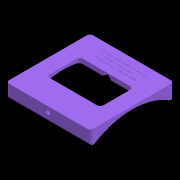
# Autodesk Inventor part: controls_flat
Saved by Autodesk Inventor 2020.2 (Build 242310000, 310)
## iProperties
Created: 2020-04-29
Part Number: controls_flat
Material: PC/ABS Plastic
Document SubType Name: Modeling
Designer: agmlego
Mass: 56.1981 g
Surface Area: 381.586 cm^2
Volume: 157.298 cm^3
Density: 0.357273 g/cm^3
Appearance: Violet
Author: agmlego
Autodesk Inventor part; units mm, degrees
(part 1 of 3)
ref_plane "YZ Plane" through (0, 0, 0) normal (1, 0, 0) x (0, 1, 0)
ref_plane "XZ Plane" through (0, 0, 0) normal (0, 1, 0) x (-1, 0, 0)
ref_plane "XY Plane" through (0, 0, 0) normal (0, 0, 1) x (1, 0, 0)
sketch "Sketch1" plane through (0, 0, 0) normal (1, 0, 0) x (0, 1, 0)
  arc A0 (87.9555, -65.2863) -> (87.9555, 65.2863) centre (0, 0) ccw
  line L0 (113.8555, 20.8363) -> (107.5375, 20.8363) construction
  line L1 (107.5375, 20.8363) -> (107.5375, -20.8363) construction
  line L2 (107.5375, -20.8363) -> (113.8555, -20.8363) construction
  line L3 (113.8555, -20.8363) -> (113.8555, 20.8363) construction
  line L4 (113.8555, 65.2863) -> (87.9555, 65.2863)
  line L5 (87.9555, -65.2863) -> (113.8555, -65.2863)
  line L6 (113.8555, -65.2863) -> (113.8555, 65.2863)
  point P0 (113.8555, 0)
  dimension "d0" = 219.075
  dimension "d1" = 113.8555
  dimension "d2" = 107.5375
  dimension "d3" = 44.45
  constraints: 14 end point, 4 parallel, 4 point on circle, 2 horizontal, 2 midpoint, 1 centre point, 1 coincident, 1 perpendicular
  measures "d0" diameter of A0
  measures "d1" distance from line of L3 A0.centre
  measures "d2" distance from line of A0.centre L1
  measures "d3" distance between parallel lines of L4 L0
extrude "Extrusion1" add sketch "Sketch1" along normal blind 130.8
sketch "Sketch2" plane through (0, 113.8555, 65.2863) normal (0, 1, 0) x (1, 0, 0)
  line L0 (25.4, 44.4498) -> (105.4, 44.4498) construction
  line L1 (105.4, 44.4498) -> (105.4, 86.1228) construction
  line L2 (105.4, 86.1228) -> (25.4, 86.1228) construction
  line L3 (25.4, 86.1228) -> (25.4, 44.4498) construction
  line L4 (0, 130.5725) -> (0, 0) construction
  circle A0 centre (28.575, 44.4498) radius 3.175 construction
  circle A1 centre (28.575, 44.4498) radius 4.953 construction
  line L5 (23.622, 39.4968) -> (107.178, 39.4968)
  line L6 (107.178, 39.4968) -> (107.178, 91.0758)
  line L7 (107.178, 91.0758) -> (23.622, 91.0758)
  line L8 (23.622, 91.0758) -> (23.622, 39.4968)
  point P0 (0, 65.2863)
  point P1 (25.4, 65.2863)
  point P2 (0, 65.2863)
  point P3 (23.622, 65.2863)
  point P4 (65.4, 91.0758)
  point P5 (65.4, 86.1228)
  dimension "d6" = 80
  dimension "d7" = 25.4
  dimension "d8" = 41.673
  dimension "d9" = 6.35
  dimension "d10" = 9.906
  constraints: 16 end point, 5 midpoint, 4 parallel, 3 tangent, 2 centre point, 2 horizontal, 2 horizontal alignment, 2 perpendicular, 1 coincident, 1 point on line, 1 vertical alignment
  measures "d6" distance of L1.end L2.end
  measures "d7" distance between parallel lines of L4 L3
  measures "d8" distance of L0.end L1.end
  measures "d9" diameter of A0
  measures "d10" diameter of A1
extrude "Extrusion2" cut sketch "Sketch2" against normal through all
fillet "Fillet1" radius 4.953 10 edges at (23.622, 110.1569, -25.7895) (23.622, 110.1569, 25.7895) (107.178, 110.1569, 25.7895) (107.178, 110.1569, -25.7895) (65.4, 87.9555, 65.2863) (65.4, 87.9555, -65.2863) (0, 100.9055, 65.2863) (0, 100.9055, -65.2863) (130.8, 100.9055, -65.2863) (130.8, 100.9055, 65.2863)
sketch "Sketch3" plane through (0, 113.8555, 65.2863) normal (0, 1, 0) x (1, 0, 0)
  line L0 (16.3484, 118.3923) -> (114.0865, 118.3923) construction
  line L1 (114.0865, 118.3923) -> (114.0865, 82.237) construction
  line L2 (114.0865, 82.237) -> (16.3484, 82.237) construction
  line L3 (16.3484, 82.237) -> (16.3484, 118.3923) construction
  spline S0 degree 2 poles (32.4092, 115.5523) (32.2458, 115.4201) (31.849, 115.3086) (31.6104, 115.3086) knots 0 0 0 1 2 2 2
  spline S1 degree 2 poles (31.6104, 115.3086) (31.3225, 115.3086) (30.8609, 115.5601) (30.5393, 115.9881) (30.3707, 116.5638) (30.3707, 116.888) knots 0 0 0 1 2 3 4 4 4
  spline S2 degree 2 poles (30.3707, 116.888) (30.3707, 117.1915) (30.5237, 117.7361) (30.8401, 118.1459) (31.3251, 118.3871) (31.6571, 118.3871) knots 0 0 0 1 2 3 4 4 4
  spline S3 degree 2 poles (31.6571, 118.3871) (31.8879, 118.3871) (32.3003, 118.2393) (32.4455, 118.1018) knots 0 0 0 1 2 2 2
  line L4 (32.4455, 118.1018) -> (32.264, 117.8865)
  spline S4 degree 2 poles (32.264, 117.8865) (32.168, 117.9514) (31.8775, 118.0473) (31.6908, 118.0473) knots 0 0 0 1 2 2 2
  spline S5 degree 2 poles (31.6908, 118.0473) (31.4444, 118.0473) (31.1047, 117.8632) (30.8868, 117.5468) (30.7883, 117.1292) (30.7883, 116.8932) knots 0 0 0 1 2 3 4 4 4
  spline S6 degree 2 poles (30.7883, 116.8932) (30.7883, 116.7557) (30.8323, 116.4653) (30.9231, 116.1878) (31.0658, 115.944) (31.2603, 115.7598) (31.5093, 115.6509) (31.6623, 115.6509) knots 0 0 0 1 2 3 4 5 6 6 6
  spline S7 degree 2 poles (31.6623, 115.6509) (31.7531, 115.6509) (31.9035, 115.6665) (32.0409, 115.7028) (32.1784, 115.7624) (32.2562, 115.8065) knots 0 0 0 1 2 3 4 4 4
  line L5 (32.2562, 115.8065) -> (32.4092, 115.5523)
  spline S8 degree 2 poles (34.2065, 115.3086) (33.8901, 115.3086) (33.387, 115.542) (33.0369, 115.9518) (32.8501, 116.5171) (32.8501, 116.8491) knots 0 0 0 1 2 3 4 4 4
  spline S9 degree 2 poles (32.8501, 116.8491) (32.8501, 117.1785) (33.0317, 117.7439) (33.3766, 118.1537) (33.8823, 118.3871) (34.2065, 118.3871) knots 0 0 0 1 2 3 4 4 4
  spline S10 degree 2 poles (34.2065, 118.3871) (34.5204, 118.3871) (35.0261, 118.1537) (35.3762, 117.7439) (35.563, 117.1785) (35.563, 116.8491) knots 0 0 0 1 2 3 4 4 4
  spline S11 degree 2 poles (35.563, 116.8491) (35.563, 116.5171) (35.3814, 115.9518) (35.0365, 115.542) (34.5307, 115.3086) (34.2065, 115.3086) knots 0 0 0 1 2 3 4 4 4
  spline S12 degree 2 poles (35.1454, 116.7869) (35.1454, 116.9451) (35.1013, 117.2563) (35.0053, 117.5364) (34.8523, 117.775) (34.6423, 117.9462) (34.3673, 118.0447) (34.1936, 118.0447) knots 0 0 0 1 2 3 4 5 6 6 6
  spline S13 degree 2 poles (34.1936, 118.0447) (33.9472, 118.0447) (33.5971, 117.8554) (33.3714, 117.5364) (33.2677, 117.1318) (33.2677, 116.9191) knots 0 0 0 1 2 3 4 4 4
  spline S14 degree 2 poles (33.2677, 116.9191) (33.2677, 116.7557) (33.3144, 116.4419) (33.4103, 116.1592) (33.5607, 115.9206) (33.7708, 115.7495) (34.0457, 115.6509) (34.2195, 115.6509) knots 0 0 0 1 2 3 4 5 6 6 6
  spline S15 degree 2 poles (34.2195, 115.6509) (34.3803, 115.6509) (34.6448, 115.7417) (34.8523, 115.8973) (35.0002, 116.1151) (35.0987, 116.3641) (35.1454, 116.6442) (35.1454, 116.7869) knots 0 0 0 1 2 3 4 5 6 6 6
  line L6 (38.019, 115.3423) -> (36.7845, 117.4067)
  line L7 (36.7845, 117.4067) -> (36.5511, 117.9851)
  line L8 (36.5511, 117.9851) -> (36.5381, 117.9851)
  line L9 (36.5381, 117.9851) -> (36.6133, 117.3497)
  line L10 (36.6133, 117.3497) -> (36.6133, 115.3423)
  line L11 (36.6133, 115.3423) -> (36.2139, 115.3423)
  line L12 (36.2139, 115.3423) -> (36.2139, 117.9306)
  line L13 (36.2139, 117.9306) -> (36.1543, 118.3534)
  line L14 (36.1543, 118.3534) -> (36.6263, 118.3923)
  line L15 (36.6263, 118.3923) -> (37.8634, 116.3174)
  line L16 (37.8634, 116.3174) -> (38.1046, 115.6872)
  line L17 (38.1046, 115.6872) -> (38.115, 115.6898)
  line L18 (38.115, 115.6898) -> (38.019, 116.3641)
  line L19 (38.019, 116.3641) -> (38.019, 118.3534)
  line L20 (38.019, 118.3534) -> (38.4107, 118.3923)
  line L21 (38.4107, 118.3923) -> (38.4107, 115.3423)
  line L22 (38.4107, 115.3423) -> (38.019, 115.3423)
  line L23 (39.8164, 115.3423) -> (39.8164, 118.0318)
  line L24 (39.8164, 118.0318) -> (38.9838, 118.0318)
  line L25 (38.9838, 118.0318) -> (38.9838, 118.3534)
  line L26 (38.9838, 118.3534) -> (41.0613, 118.3534)
  line L27 (41.0613, 118.3534) -> (41.0613, 118.0318)
  line L28 (41.0613, 118.0318) -> (40.2391, 118.0318)
  line L29 (40.2391, 118.0318) -> (40.2391, 115.3423)
  line L30 (40.2391, 115.3423) -> (39.8164, 115.3423)
  line L31 (42.0364, 116.5742) -> (42.0364, 115.3423)
  line L32 (42.0364, 115.3423) -> (41.6137, 115.3423)
  line L33 (41.6137, 115.3423) -> (41.6137, 117.9306)
  line L34 (41.6137, 117.9306) -> (41.5437, 118.3326)
  spline S16 degree 2 poles (41.5437, 118.3326) (41.6085, 118.3404) (41.7952, 118.356) (42.0001, 118.3689) (42.2024, 118.3767) (42.2906, 118.3767) knots 0 0 0 1 2 3 4 4 4
  spline S17 degree 2 poles (42.2906, 118.3767) (42.5422, 118.3767) (42.9597, 118.2704) (43.258, 118.0629) (43.4214, 117.7517) (43.4214, 117.5468) knots 0 0 0 1 2 3 4 4 4
  spline S18 degree 2 poles (43.4214, 117.5468) (43.4214, 117.3367) (43.2917, 117.0151) (43.0531, 116.7895) (42.7263, 116.6468) (42.5318, 116.6131) knots 0 0 0 1 2 3 4 4 4
  line L35 (42.5318, 116.6131) -> (42.8171, 116.5327)
  line L36 (42.8171, 116.5327) -> (43.7067, 115.3423)
  line L37 (43.7067, 115.3423) -> (43.258, 115.3423)
  line L38 (43.258, 115.3423) -> (42.371, 116.5353)
  spline S19 degree 2 poles (42.371, 116.5353) (42.3477, 116.5638) (42.2932, 116.5742) (42.2776, 116.5742) knots 0 0 0 1 2 2 2
  line L39 (42.2776, 116.5742) -> (42.0364, 116.5742)
  line L40 (42.0364, 117.6427) -> (42.0364, 116.8776)
  line L41 (42.0364, 116.8776) -> (42.3321, 116.8776)
  spline S20 degree 2 poles (42.3321, 116.8776) (42.5162, 116.8776) (42.7834, 116.9788) (42.9597, 117.1552) (43.0479, 117.386) (43.0479, 117.5157) knots 0 0 0 1 2 3 4 4 4
  spline S21 degree 2 poles (43.0479, 117.5157) (43.0479, 117.6868) (42.9208, 117.9125) (42.7159, 118.0473) (42.4644, 118.1018) (42.3399, 118.1018) knots 0 0 0 1 2 3 4 4 4
  spline S22 degree 2 poles (42.3399, 118.1018) (42.2984, 118.1018) (42.2076, 118.0992) (42.1142, 118.0966) (42.0286, 118.0836) (41.9975, 118.0785) knots 0 0 0 1 2 3 4 4 4
  line L42 (41.9975, 118.0785) -> (42.0364, 117.6427)
  spline S23 degree 2 poles (45.4469, 115.3086) (45.1305, 115.3086) (44.6274, 115.542) (44.2772, 115.9518) (44.0905, 116.5171) (44.0905, 116.8491) knots 0 0 0 1 2 3 4 4 4
  spline S24 degree 2 poles (44.0905, 116.8491) (44.0905, 117.1785) (44.2721, 117.7439) (44.617, 118.1537) (45.1227, 118.3871) (45.4469, 118.3871) knots 0 0 0 1 2 3 4 4 4
  spline S25 degree 2 poles (45.4469, 118.3871) (45.7607, 118.3871) (46.2665, 118.1537) (46.6166, 117.7439) (46.8034, 117.1785) (46.8034, 116.8491) knots 0 0 0 1 2 3 4 4 4
  spline S26 degree 2 poles (46.8034, 116.8491) (46.8034, 116.5171) (46.6218, 115.9518) (46.2769, 115.542) (45.7711, 115.3086) (45.4469, 115.3086) knots 0 0 0 1 2 3 4 4 4
  spline S27 degree 2 poles (46.3858, 116.7869) (46.3858, 116.9451) (46.3417, 117.2563) (46.2457, 117.5364) (46.0927, 117.775) (45.8826, 117.9462) (45.6077, 118.0447) (45.434, 118.0447) knots 0 0 0 1 2 3 4 5 6 6 6
  spline S28 degree 2 poles (45.434, 118.0447) (45.1876, 118.0447) (44.8374, 117.8554) (44.6118, 117.5364) (44.5081, 117.1318) (44.5081, 116.9191) knots 0 0 0 1 2 3 4 4 4
  spline S29 degree 2 poles (44.5081, 116.9191) (44.5081, 116.7557) (44.5548, 116.4419) (44.6507, 116.1592) (44.8011, 115.9206) (45.0112, 115.7495) (45.2861, 115.6509) (45.4599, 115.6509) knots 0 0 0 1 2 3 4 5 6 6 6
  spline S30 degree 2 poles (45.4599, 115.6509) (45.6207, 115.6509) (45.8852, 115.7417) (46.0927, 115.8973) (46.2406, 116.1151) (46.3391, 116.3641) (46.3858, 116.6442) (46.3858, 116.7869) knots 0 0 0 1 2 3 4 5 6 6 6
  line L43 (47.8356, 115.6639) -> (49.1401, 115.6639)
  line L44 (49.1401, 115.6639) -> (49.1012, 115.3423)
  line L45 (49.1012, 115.3423) -> (47.3947, 115.3423)
  line L46 (47.3947, 115.3423) -> (47.4336, 115.7443)
  line L47 (47.4336, 115.7443) -> (47.4336, 117.9306)
  line L48 (47.4336, 117.9306) -> (47.3739, 118.3534)
  line L49 (47.3739, 118.3534) -> (47.8563, 118.3923)
  line L50 (47.8563, 118.3923) -> (47.8563, 116.0244)
  line L51 (47.8563, 116.0244) -> (47.8356, 115.6639)
  spline S31 degree 2 poles (51.0075, 117.8995) (50.87, 117.9799) (50.6184, 118.0551) (50.4654, 118.0551) knots 0 0 0 1 2 2 2
  spline S32 degree 2 poles (50.4654, 118.0551) (50.3565, 118.0551) (50.149, 118.011) (49.9908, 117.9125) (49.8923, 117.7543) (49.8923, 117.6401) knots 0 0 0 1 2 3 4 4 4
  spline S33 degree 2 poles (49.8923, 117.6401) (49.8923, 117.5286) (50.0116, 117.3626) (50.2061, 117.233) (50.4576, 117.1214) (50.7196, 116.9995) (50.9712, 116.8543) (51.1657, 116.6546) (51.285, 116.3901) (51.285, 116.2085) knots 0 0 0 1 2 3 4 5 6 7 8 8 8
  spline S34 degree 2 poles (51.285, 116.2085) (51.285, 116.0607) (51.2046, 115.8091) (51.0619, 115.6094) (50.8648, 115.459) (50.6314, 115.3578) (50.3747, 115.3086) (50.2398, 115.3086) knots 0 0 0 1 2 3 4 5 6 6 6
  spline S35 degree 2 poles (50.2398, 115.3086) (49.7704, 115.3163) (49.4228, 115.5316) knots 0 0 0 1 1 1
  line L52 (49.4228, 115.5316) -> (49.607, 115.8324)
  spline S36 degree 2 poles (49.607, 115.8324) (49.6459, 115.8065) (49.7781, 115.7417) (49.9389, 115.6794) (50.1179, 115.6405) (50.2113, 115.6405) knots 0 0 0 1 2 3 4 4 4
  spline S37 degree 2 poles (50.2113, 115.6405) (50.3357, 115.6405) (50.5744, 115.7028) (50.7611, 115.8324) (50.8752, 116.0347) (50.8752, 116.1722) knots 0 0 0 1 2 3 4 4 4
  spline S38 degree 2 poles (50.8752, 116.1722) (50.8752, 116.3019) (50.7559, 116.4964) (50.5614, 116.652) (50.3098, 116.7765) (50.0479, 116.901) (49.7963, 117.0358) (49.6018, 117.2096) (49.4825, 117.4327) (49.4825, 117.5831) knots 0 0 0 1 2 3 4 5 6 7 8 8 8
  spline S39 degree 2 poles (49.4825, 117.5831) (49.4825, 117.7776) (49.6433, 118.0759) (49.9052, 118.2807) (50.2398, 118.3871) (50.411, 118.3871) knots 0 0 0 1 2 3 4 4 4
  spline S40 degree 2 poles (50.411, 118.3871) (50.8389, 118.3871) (51.202, 118.1459) knots 0 0 0 1 1 1
  line L53 (51.202, 118.1459) -> (51.0075, 117.8995)
  line L54 (53.6762, 115.3423) -> (53.2535, 115.3423)
  line L55 (53.2535, 115.3423) -> (53.2535, 117.9306)
  line L56 (53.2535, 117.9306) -> (53.1938, 118.3534)
  line L57 (53.1938, 118.3534) -> (54.9704, 118.3534)
  line L58 (54.9704, 118.3534) -> (54.9315, 118.0318)
  line L59 (54.9315, 118.0318) -> (53.6373, 118.0318)
  line L60 (53.6373, 118.0318) -> (53.6762, 117.6505)
  line L61 (53.6762, 117.6505) -> (53.6762, 117.1188)
  line L62 (53.6762, 117.1188) -> (54.7603, 117.1188)
  line L63 (54.7603, 117.1188) -> (54.7603, 116.831)
  line L64 (54.7603, 116.831) -> (53.6762, 116.831)
  line L65 (53.6762, 116.831) -> (53.6762, 115.3423)
  line L66 (55.8626, 115.6639) -> (57.1671, 115.6639)
  line L67 (57.1671, 115.6639) -> (57.1282, 115.3423)
  line L68 (57.1282, 115.3423) -> (55.4217, 115.3423)
  line L69 (55.4217, 115.3423) -> (55.4606, 115.7443)
  line L70 (55.4606, 115.7443) -> (55.4606, 117.9306)
  line L71 (55.4606, 117.9306) -> (55.4009, 118.3534)
  line L72 (55.4009, 118.3534) -> (55.8833, 118.3923)
  line L73 (55.8833, 118.3923) -> (55.8833, 116.0244)
  line L74 (55.8833, 116.0244) -> (55.8626, 115.6639)
  line L75 (57.4109, 115.3423) -> (58.2616, 117.9514)
  line L76 (58.2616, 117.9514) -> (58.3316, 118.3534)
  line L77 (58.3316, 118.3534) -> (58.7673, 118.3923)
  line L78 (58.7673, 118.3923) -> (59.7659, 115.3423)
  line L79 (59.7659, 115.3423) -> (59.3639, 115.3423)
  line L80 (59.3639, 115.3423) -> (59.0656, 116.2448)
  line L81 (59.0656, 116.2448) -> (58.0723, 116.2448)
  line L82 (58.0723, 116.2448) -> (57.7792, 115.3423)
  line L83 (57.7792, 115.3423) -> (57.4109, 115.3423)
  line L84 (58.5702, 118.0707) -> (58.4976, 117.5494)
  line L85 (58.4976, 117.5494) -> (58.1708, 116.5457)
  line L86 (58.1708, 116.5457) -> (58.9696, 116.5457)
  line L87 (58.9696, 116.5457) -> (58.6403, 117.5494)
  line L88 (58.6403, 117.5494) -> (58.5702, 118.0707)
  line L89 (60.8889, 115.3423) -> (60.8889, 118.0318)
  line L90 (60.8889, 118.0318) -> (60.0563, 118.0318)
  line L91 (60.0563, 118.0318) -> (60.0563, 118.3534)
  line L92 (60.0563, 118.3534) -> (62.1338, 118.3534)
  line L93 (62.1338, 118.3534) -> (62.1338, 118.0318)
  line L94 (62.1338, 118.0318) -> (61.3116, 118.0318)
  line L95 (61.3116, 118.0318) -> (61.3116, 115.3423)
  line L96 (61.3116, 115.3423) -> (60.8889, 115.3423)
  spline S41 degree 2 poles (64.9374, 118.3871) (65.1215, 118.3871) (65.4353, 118.2859) (65.661, 118.0992) (65.7906, 117.8295) (65.7906, 117.6609) knots 0 0 0 1 2 3 4 4 4
  spline S42 degree 2 poles (65.7906, 117.6609) (65.7906, 117.5416) (65.7206, 117.3574) (65.5987, 117.2122) (65.4405, 117.0929) (65.3523, 117.041) knots 0 0 0 1 2 3 4 4 4
  spline S43 degree 2 poles (65.3523, 117.041) (65.5002, 116.9736) (65.7362, 116.8024) (65.8996, 116.5898) (65.9852, 116.3252) (65.9852, 116.1644) knots 0 0 0 1 2 3 4 4 4
  spline S44 degree 2 poles (65.9852, 116.1644) (65.9852, 115.944) (65.8088, 115.6198) (65.5183, 115.4097) (65.1448, 115.3086) (64.9503, 115.3086) knots 0 0 0 1 2 3 4 4 4
  spline S45 degree 2 poles (64.9503, 115.3086) (64.7584, 115.3086) (64.4057, 115.4227) (64.136, 115.6457) (63.97, 115.9777) (63.97, 116.1929) knots 0 0 0 1 2 3 4 4 4
  spline S46 degree 2 poles (63.97, 116.1929) (63.97, 116.3537) (64.0633, 116.6157) (64.2241, 116.8232) (64.4446, 116.9866) (64.5717, 117.0488) knots 0 0 0 1 2 3 4 4 4
  spline S47 degree 2 poles (64.5717, 117.0488) (64.4783, 117.1059) (64.3149, 117.2304) (64.193, 117.373) (64.123, 117.539) (64.123, 117.6376) knots 0 0 0 1 2 3 4 4 4
  spline S48 degree 2 poles (64.123, 117.6376) (64.123, 117.8321) (64.2786, 118.1174) (64.5198, 118.2989) (64.8051, 118.3871) (64.9374, 118.3871) knots 0 0 0 1 2 3 4 4 4
  spline S49 degree 2 poles (64.914, 116.8673) (64.7869, 116.8154) (64.5846, 116.6831) (64.442, 116.5171) (64.3642, 116.3097) (64.3642, 116.1748) knots 0 0 0 1 2 3 4 4 4
  spline S50 degree 2 poles (64.3642, 116.1748) (64.3642, 116.0529) (64.4627, 115.8558) (64.6261, 115.7131) (64.8388, 115.6379) (64.9503, 115.6379) knots 0 0 0 1 2 3 4 4 4
  spline S51 degree 2 poles (64.9503, 115.6379) (65.08, 115.6379) (65.3108, 115.708) (65.4846, 115.8454) (65.5857, 116.0451) (65.5857, 116.1748) knots 0 0 0 1 2 3 4 4 4
  spline S52 degree 2 poles (65.5857, 116.1748) (65.5857, 116.3097) (65.4664, 116.5223) (65.2771, 116.6883) (65.0385, 116.8154) (64.914, 116.8673) knots 0 0 0 1 2 3 4 4 4
  spline S53 degree 2 poles (64.9996, 117.1941) (65.1838, 117.277) (65.4042, 117.5105) (65.4042, 117.6765) knots 0 0 0 1 2 2 2
  spline S54 degree 2 poles (65.4042, 117.6765) (65.4042, 117.7776) (65.3212, 117.9202) (65.1967, 118.0136) (65.0437, 118.0551) (64.9763, 118.0551) knots 0 0 0 1 2 3 4 4 4
  spline S55 degree 2 poles (64.9763, 118.0551) (64.8855, 118.0551) (64.7169, 118.0006) (64.5872, 117.8995) (64.5094, 117.7646) (64.5094, 117.6842) knots 0 0 0 1 2 3 4 4 4
  spline S56 degree 2 poles (64.5094, 117.6842) (64.5094, 117.5909) (64.5872, 117.4508) (64.7221, 117.3367) (64.9011, 117.2381) (64.9996, 117.1941) knots 0 0 0 1 2 3 4 4 4
  spline S57 degree 2 poles (67.5257, 115.3086) (67.3545, 115.3086) (67.0693, 115.4382) (66.8436, 115.6639) (66.6724, 115.9647) (66.5583, 116.3071) (66.5013, 116.6702) (66.5013, 116.8491) knots 0 0 0 1 2 3 4 5 6 6 6
  spline S58 degree 2 poles (66.5013, 116.8491) (66.5013, 117.0281) (66.5505, 117.3989) (66.6543, 117.7387) (66.8177, 118.037) (67.0433, 118.2574) (67.339, 118.3871) (67.5257, 118.3871) knots 0 0 0 1 2 3 4 5 6 6 6
  spline S59 degree 2 poles (67.5257, 118.3871) (67.6969, 118.3871) (67.9822, 118.2574) (68.2078, 118.0318) (68.379, 117.7309) (68.4931, 117.3886) (68.5502, 117.0229) (68.5502, 116.8491) knots 0 0 0 1 2 3 4 5 6 6 6
  spline S60 degree 2 poles (68.5502, 116.8491) (68.5502, 116.6676) (68.5009, 116.2967) (68.3971, 115.9569) (68.2338, 115.6587) (68.0081, 115.4382) (67.7099, 115.3086) (67.5257, 115.3086) knots 0 0 0 1 2 3 4 5 6 6 6
  spline S61 degree 2 poles (66.9188, 116.9347) (66.9188, 116.818) (66.9344, 116.5379) (66.9837, 116.2552) (67.0693, 115.9907) (67.2067, 115.7832) (67.4064, 115.6587) (67.5413, 115.6587) knots 0 0 0 1 2 3 4 5 6 6 6
  spline S62 degree 2 poles (67.5413, 115.6587) (67.6632, 115.6587) (67.8473, 115.752) (67.9796, 115.9154) (68.0626, 116.1307) (68.1119, 116.3745) (68.1326, 116.6364) (68.1326, 116.7609) knots 0 0 0 1 2 3 4 5 6 6 6
  spline S63 degree 2 poles (68.1326, 116.7609) (68.1326, 116.8776) (68.117, 117.1577) (68.0678, 117.4378) (67.9822, 117.705) (67.8447, 117.9099) (67.645, 118.0344) (67.5102, 118.0344) knots 0 0 0 1 2 3 4 5 6 6 6
  spline S64 degree 2 poles (67.5102, 118.0344) (67.3883, 118.0344) (67.2041, 117.941) (67.0718, 117.7802) (66.9889, 117.5623) (66.9396, 117.3185) (66.9188, 117.0592) (66.9188, 116.9347) knots 0 0 0 1 2 3 4 5 6 6 6
  line L97 (69.7121, 115.3423) -> (69.3308, 115.3423)
  line L98 (69.3308, 115.3423) -> (69.3308, 117.552)
  line L99 (69.3308, 117.552) -> (69.7121, 117.5909)
  line L100 (69.7121, 117.5909) -> (69.7121, 117.2226)
  line L101 (69.7121, 117.2226) -> (69.834, 117.4378)
  spline S65 degree 2 poles (69.834, 117.4378) (69.8703, 117.4638) (69.9792, 117.5157) (70.1167, 117.5572) (70.2723, 117.5857) (70.3553, 117.5857) knots 0 0 0 1 2 3 4 4 4
  spline S66 degree 2 poles (70.3553, 117.5857) (70.5783, 117.5857) (70.861, 117.3652) (70.9025, 117.1966) knots 0 0 0 1 2 2 2
  line L102 (70.9025, 117.1966) -> (71.0555, 117.4301)
  spline S67 degree 2 poles (71.0555, 117.4301) (71.1255, 117.4871) (71.3823, 117.5857) (71.5483, 117.5857) knots 0 0 0 1 2 2 2
  spline S68 degree 2 poles (71.5483, 117.5857) (71.7013, 117.5857) (71.9192, 117.4845) (72.0566, 117.29) (72.1215, 117.0177) (72.1215, 116.8491) knots 0 0 0 1 2 3 4 4 4
  line L103 (72.1215, 116.8491) -> (72.1215, 115.3423)
  line L104 (72.1215, 115.3423) -> (71.7402, 115.3423)
  line L105 (71.7402, 115.3423) -> (71.7402, 116.8284)
  spline S69 degree 2 poles (71.7402, 116.8284) (71.7402, 116.9373) (71.7091, 117.1007) (71.6365, 117.2096) (71.512, 117.2641) (71.4186, 117.2641) knots 0 0 0 1 2 3 4 4 4
  spline S70 degree 2 poles (71.4186, 117.2641) (71.3616, 117.2641) (71.2345, 117.2252) (71.1048, 117.1577) (70.9829, 117.0722) (70.9284, 117.0281) knots 0 0 0 1 2 3 4 4 4
  spline S71 degree 2 poles (70.9284, 117.0281) (70.9336, 116.9684) (70.9362, 116.8906) (70.9362, 116.8284) knots 0 0 0 1 2 2 2
  line L106 (70.9362, 116.8284) -> (70.9362, 115.3423)
  line L107 (70.9362, 115.3423) -> (70.555, 115.3423)
  line L108 (70.555, 115.3423) -> (70.555, 116.8284)
  spline S72 degree 2 poles (70.555, 116.8284) (70.555, 117.0462) (70.4097, 117.2641) (70.223, 117.2641) knots 0 0 0 1 2 2 2
  spline S73 degree 2 poles (70.223, 117.2641) (70.1633, 117.2641) (70.0259, 117.2278) (69.8936, 117.1629) (69.7639, 117.0825) (69.7121, 117.0384) knots 0 0 0 1 2 3 4 4 4
  line L109 (69.7121, 117.0384) -> (69.7121, 115.3423)
  line L110 (73.3249, 115.3423) -> (72.9436, 115.3423)
  line L111 (72.9436, 115.3423) -> (72.9436, 117.552)
  line L112 (72.9436, 117.552) -> (73.3249, 117.5909)
  line L113 (73.3249, 117.5909) -> (73.3249, 117.2226)
  line L114 (73.3249, 117.2226) -> (73.4468, 117.4378)
  spline S74 degree 2 poles (73.4468, 117.4378) (73.4831, 117.4638) (73.592, 117.5157) (73.7295, 117.5572) (73.8851, 117.5857) (73.9681, 117.5857) knots 0 0 0 1 2 3 4 4 4
  spline S75 degree 2 poles (73.9681, 117.5857) (74.1911, 117.5857) (74.4738, 117.3652) (74.5153, 117.1966) knots 0 0 0 1 2 2 2
  line L115 (74.5153, 117.1966) -> (74.6683, 117.4301)
  spline S76 degree 2 poles (74.6683, 117.4301) (74.7383, 117.4871) (74.9951, 117.5857) (75.1611, 117.5857) knots 0 0 0 1 2 2 2
  spline S77 degree 2 poles (75.1611, 117.5857) (75.3141, 117.5857) (75.532, 117.4845) (75.6694, 117.29) (75.7343, 117.0177) (75.7343, 116.8491) knots 0 0 0 1 2 3 4 4 4
  line L116 (75.7343, 116.8491) -> (75.7343, 115.3423)
  line L117 (75.7343, 115.3423) -> (75.353, 115.3423)
  line L118 (75.353, 115.3423) -> (75.353, 116.8284)
  spline S78 degree 2 poles (75.353, 116.8284) (75.353, 116.9373) (75.3219, 117.1007) (75.2493, 117.2096) (75.1248, 117.2641) (75.0314, 117.2641) knots 0 0 0 1 2 3 4 4 4
  spline S79 degree 2 poles (75.0314, 117.2641) (74.9744, 117.2641) (74.8473, 117.2252) (74.7176, 117.1577) (74.5957, 117.0722) (74.5412, 117.0281) knots 0 0 0 1 2 3 4 4 4
  spline S80 degree 2 poles (74.5412, 117.0281) (74.5464, 116.9684) (74.549, 116.8906) (74.549, 116.8284) knots 0 0 0 1 2 2 2
  line L119 (74.549, 116.8284) -> (74.549, 115.3423)
  line L120 (74.549, 115.3423) -> (74.1678, 115.3423)
  line L121 (74.1678, 115.3423) -> (74.1678, 116.8284)
  spline S81 degree 2 poles (74.1678, 116.8284) (74.1678, 117.0462) (74.0225, 117.2641) (73.8358, 117.2641) knots 0 0 0 1 2 2 2
  spline S82 degree 2 poles (73.8358, 117.2641) (73.7761, 117.2641) (73.6387, 117.2278) (73.5064, 117.1629) (73.3767, 117.0825) (73.3249, 117.0384) knots 0 0 0 1 2 3 4 4 4
  line L122 (73.3249, 117.0384) -> (73.3249, 115.3423)
  line L123 (79.3107, 118.3534) -> (79.6272, 118.3534)
  line L124 (79.6272, 118.3534) -> (80.1459, 116.2656)
  line L125 (80.1459, 116.2656) -> (80.2755, 115.542)
  line L126 (80.2755, 115.542) -> (80.2833, 115.542)
  line L127 (80.2833, 115.542) -> (80.3274, 116.2656)
  line L128 (80.3274, 116.2656) -> (80.8513, 118.3534)
  line L129 (80.8513, 118.3534) -> (81.2014, 118.3534)
  line L130 (81.2014, 118.3534) -> (80.4493, 115.3423)
  line L131 (80.4493, 115.3423) -> (79.9851, 115.3423)
  line L132 (79.9851, 115.3423) -> (79.5416, 117.1188)
  line L133 (79.5416, 117.1188) -> (79.4845, 117.8373)
  line L134 (79.4845, 117.8373) -> (79.3548, 117.1188)
  line L135 (79.3548, 117.1188) -> (78.9113, 115.3423)
  line L136 (78.9113, 115.3423) -> (78.4445, 115.3423)
  line L137 (78.4445, 115.3423) -> (77.695, 118.3534)
  line L138 (77.695, 118.3534) -> (78.0788, 118.3923)
  line L139 (78.0788, 118.3923) -> (78.6079, 116.2656)
  line L140 (78.6079, 116.2656) -> (78.7376, 115.542)
  line L141 (78.7376, 115.542) -> (78.7454, 115.542)
  line L142 (78.7454, 115.542) -> (78.7894, 116.2656)
  line L143 (78.7894, 116.2656) -> (79.3107, 118.3534)
  line L144 (84.49, 115.3423) -> (83.9506, 116.11)
  line L145 (83.9506, 116.11) -> (83.8624, 116.346)
  line L146 (83.8624, 116.346) -> (83.7716, 116.11)
  line L147 (83.7716, 116.11) -> (83.2322, 115.3423)
  line L148 (83.2322, 115.3423) -> (82.8328, 115.3423)
  line L149 (82.8328, 115.3423) -> (83.6601, 116.5223)
  line L150 (83.6601, 116.5223) -> (82.9417, 117.552)
  line L151 (82.9417, 117.552) -> (83.3644, 117.5857)
  line L152 (83.3644, 117.5857) -> (83.8365, 116.9114)
  line L153 (83.8365, 116.9114) -> (83.9169, 116.6883)
  line L154 (83.9169, 116.6883) -> (83.9921, 116.9114)
  line L155 (83.9921, 116.9114) -> (84.4434, 117.552)
  line L156 (84.4434, 117.552) -> (84.8661, 117.5857)
  line L157 (84.8661, 117.5857) -> (84.1166, 116.512)
  line L158 (84.1166, 116.512) -> (84.9413, 115.3423)
  line L159 (84.9413, 115.3423) -> (84.49, 115.3423)
  line L160 (86.6997, 115.3423) -> (86.6997, 115.6794)
  spline S83 degree 2 poles (86.6997, 115.6794) (86.7957, 115.8324) (87.0187, 116.1281) (87.2444, 116.403) (87.4648, 116.6494) (87.5582, 116.7506) knots 0 0 0 1 2 3 4 4 4
  spline S84 degree 2 poles (87.5582, 116.7506) (87.6593, 116.8647) (87.8435, 117.0618) (87.9861, 117.2589) (88.0691, 117.4612) (88.0691, 117.5805) knots 0 0 0 1 2 3 4 4 4
  spline S85 degree 2 poles (88.0691, 117.5805) (88.0691, 117.6765) (87.9965, 117.8476) (87.8668, 117.9721) (87.6853, 118.0473) (87.5764, 118.0473) knots 0 0 0 1 2 3 4 4 4
  spline S86 degree 2 poles (87.5764, 118.0473) (87.4545, 118.0473) (87.2755, 117.9799) (87.1406, 117.8736) (87.0421, 117.7387) (87.0006, 117.6687) knots 0 0 0 1 2 3 4 4 4
  line L161 (87.0006, 117.6687) -> (86.7179, 117.7906)
  spline S87 degree 2 poles (86.7179, 117.7906) (86.7698, 117.9202) (86.9332, 118.1407) (87.1536, 118.2989) (87.4337, 118.3871) (87.6075, 118.3871) knots 0 0 0 1 2 3 4 4 4
  spline S88 degree 2 poles (87.6075, 118.3871) (87.8098, 118.3871) (88.1262, 118.2418) (88.3466, 118.0084) (88.4607, 117.7102) (88.4607, 117.5572) knots 0 0 0 1 2 3 4 4 4
  spline S89 degree 2 poles (88.4607, 117.5572) (88.4607, 117.4041) (88.3466, 117.124) (88.1755, 116.8751) (87.9784, 116.652) (87.898, 116.556) knots 0 0 0 1 2 3 4 4 4
  spline S90 degree 2 poles (87.898, 116.556) (87.7916, 116.4341) (87.5841, 116.1981) (87.3922, 115.9699) (87.2288, 115.7598) (87.1692, 115.6639) knots 0 0 0 1 2 3 4 4 4
  line L162 (87.1692, 115.6639) -> (88.5126, 115.6639)
  line L163 (88.5126, 115.6639) -> (88.5126, 115.3423)
  line L164 (88.5126, 115.3423) -> (86.6997, 115.3423)
  line L165 (89.786, 115.3423) -> (89.4048, 115.3423)
  line L166 (89.4048, 115.3423) -> (89.4048, 117.552)
  line L167 (89.4048, 117.552) -> (89.786, 117.5909)
  line L168 (89.786, 117.5909) -> (89.786, 117.2226)
  line L169 (89.786, 117.2226) -> (89.9079, 117.4378)
  spline S91 degree 2 poles (89.9079, 117.4378) (89.9443, 117.4638) (90.0532, 117.5157) (90.1906, 117.5572) (90.3463, 117.5857) (90.4292, 117.5857) knots 0 0 0 1 2 3 4 4 4
  spline S92 degree 2 poles (90.4292, 117.5857) (90.6523, 117.5857) (90.935, 117.3652) (90.9765, 117.1966) knots 0 0 0 1 2 2 2
  line L170 (90.9765, 117.1966) -> (91.1295, 117.4301)
  spline S93 degree 2 poles (91.1295, 117.4301) (91.1995, 117.4871) (91.4563, 117.5857) (91.6223, 117.5857) knots 0 0 0 1 2 2 2
  spline S94 degree 2 poles (91.6223, 117.5857) (91.7753, 117.5857) (91.9931, 117.4845) (92.1306, 117.29) (92.1954, 117.0177) (92.1954, 116.8491) knots 0 0 0 1 2 3 4 4 4
  line L171 (92.1954, 116.8491) -> (92.1954, 115.3423)
  line L172 (92.1954, 115.3423) -> (91.8142, 115.3423)
  line L173 (91.8142, 115.3423) -> (91.8142, 116.8284)
  spline S95 degree 2 poles (91.8142, 116.8284) (91.8142, 116.9373) (91.7831, 117.1007) (91.7105, 117.2096) (91.586, 117.2641) (91.4926, 117.2641) knots 0 0 0 1 2 3 4 4 4
  spline S96 degree 2 poles (91.4926, 117.2641) (91.4355, 117.2641) (91.3085, 117.2252) (91.1788, 117.1577) (91.0569, 117.0722) (91.0024, 117.0281) knots 0 0 0 1 2 3 4 4 4
  spline S97 degree 2 poles (91.0024, 117.0281) (91.0076, 116.9684) (91.0102, 116.8906) (91.0102, 116.8284) knots 0 0 0 1 2 2 2
  line L174 (91.0102, 116.8284) -> (91.0102, 115.3423)
  line L175 (91.0102, 115.3423) -> (90.6289, 115.3423)
  line L176 (90.6289, 115.3423) -> (90.6289, 116.8284)
  spline S98 degree 2 poles (90.6289, 116.8284) (90.6289, 117.0462) (90.4837, 117.2641) (90.297, 117.2641) knots 0 0 0 1 2 2 2
  spline S99 degree 2 poles (90.297, 117.2641) (90.2373, 117.2641) (90.0999, 117.2278) (89.9676, 117.1629) (89.8379, 117.0825) (89.786, 117.0384) knots 0 0 0 1 2 3 4 4 4
  line L177 (89.786, 117.0384) -> (89.786, 115.3423)
  line L178 (93.3988, 115.3423) -> (93.0176, 115.3423)
  line L179 (93.0176, 115.3423) -> (93.0176, 117.552)
  line L180 (93.0176, 117.552) -> (93.3988, 117.5909)
  line L181 (93.3988, 117.5909) -> (93.3988, 117.2226)
  line L182 (93.3988, 117.2226) -> (93.5207, 117.4378)
  spline S100 degree 2 poles (93.5207, 117.4378) (93.5571, 117.4638) (93.666, 117.5157) (93.8034, 117.5572) (93.959, 117.5857) (94.042, 117.5857) knots 0 0 0 1 2 3 4 4 4
  spline S101 degree 2 poles (94.042, 117.5857) (94.2651, 117.5857) (94.5478, 117.3652) (94.5893, 117.1966) knots 0 0 0 1 2 2 2
  line L183 (94.5893, 117.1966) -> (94.7423, 117.4301)
  spline S102 degree 2 poles (94.7423, 117.4301) (94.8123, 117.4871) (95.0691, 117.5857) (95.2351, 117.5857) knots 0 0 0 1 2 2 2
  spline S103 degree 2 poles (95.2351, 117.5857) (95.3881, 117.5857) (95.6059, 117.4845) (95.7434, 117.29) (95.8082, 117.0177) (95.8082, 116.8491) knots 0 0 0 1 2 3 4 4 4
  line L184 (95.8082, 116.8491) -> (95.8082, 115.3423)
  line L185 (95.8082, 115.3423) -> (95.427, 115.3423)
  line L186 (95.427, 115.3423) -> (95.427, 116.8284)
  spline S104 degree 2 poles (95.427, 116.8284) (95.427, 116.9373) (95.3959, 117.1007) (95.3232, 117.2096) (95.1988, 117.2641) (95.1054, 117.2641) knots 0 0 0 1 2 3 4 4 4
  spline S105 degree 2 poles (95.1054, 117.2641) (95.0483, 117.2641) (94.9213, 117.2252) (94.7916, 117.1577) (94.6697, 117.0722) (94.6152, 117.0281) knots 0 0 0 1 2 3 4 4 4
  spline S106 degree 2 poles (94.6152, 117.0281) (94.6204, 116.9684) (94.623, 116.8906) (94.623, 116.8284) knots 0 0 0 1 2 2 2
  line L187 (94.623, 116.8284) -> (94.623, 115.3423)
  line L188 (94.623, 115.3423) -> (94.2417, 115.3423)
  line L189 (94.2417, 115.3423) -> (94.2417, 116.8284)
  spline S107 degree 2 poles (94.2417, 116.8284) (94.2417, 117.0462) (94.0965, 117.2641) (93.9098, 117.2641) knots 0 0 0 1 2 2 2
  spline S108 degree 2 poles (93.9098, 117.2641) (93.8501, 117.2641) (93.7127, 117.2278) (93.5804, 117.1629) (93.4507, 117.0825) (93.3988, 117.0384) knots 0 0 0 1 2 3 4 4 4
  line L190 (93.3988, 117.0384) -> (93.3988, 115.3423)
  spline S109 degree 2 poles (97.9764, 118.3534) (98.0387, 118.3586) (98.2099, 118.3689) (98.394, 118.3741) (98.573, 118.3767) (98.6378, 118.3767) knots 0 0 0 1 2 3 4 4 4
  spline S110 degree 2 poles (98.6378, 118.3767) (98.9568, 118.3767) (99.5014, 118.2211) (99.8982, 117.8787) (100.1239, 117.3445) (100.1239, 116.9684) knots 0 0 0 1 2 3 4 4 4
  spline S111 degree 2 poles (100.1239, 116.9684) (100.1239, 116.6753) (100.0124, 116.2085) (99.8127, 115.8454) (99.5326, 115.5861) (99.198, 115.4201) (98.8219, 115.3423) (98.6196, 115.3423) knots 0 0 0 1 2 3 4 5 6 6 6
  line L191 (98.6196, 115.3423) -> (98.0361, 115.3423)
  line L192 (98.0361, 115.3423) -> (98.0361, 117.9306)
  line L193 (98.0361, 117.9306) -> (97.9764, 118.3534)
  line L194 (98.4588, 117.6531) -> (98.4588, 115.6639)
  line L195 (98.4588, 115.6639) -> (98.4977, 115.6639)
  spline S112 degree 2 poles (98.4977, 115.6639) (98.7882, 115.6639) (99.1954, 115.7832) (99.4599, 115.9829) (99.6104, 116.2422) (99.6856, 116.5197) (99.7011, 116.7921) (99.7011, 116.9088) knots 0 0 0 1 2 3 4 5 6 6 6
  spline S113 degree 2 poles (99.7011, 116.9088) (99.7011, 117.1655) (99.613, 117.5935) (99.3769, 117.8995) (98.9542, 118.0707) (98.6222, 118.0707) knots 0 0 0 1 2 3 4 4 4
  spline S114 degree 2 poles (98.6222, 118.0707) (98.5885, 118.0707) (98.5159, 118.0681) (98.4848, 118.0629) knots 0 0 0 1 2 2 2
  spline S115 degree 2 poles (98.4848, 118.0629) (98.4485, 118.0603) (98.4096, 118.0551) knots 0 0 0 1 1 1
  line L196 (98.4096, 118.0551) -> (98.4588, 117.6531)
  spline S116 degree 2 poles (42.987, 110.987) (42.987, 111.166) (43.0233, 111.4746) (43.1452, 111.7028) (43.3838, 111.8299) (43.5887, 111.8299) knots 0 0 0 1 2 3 4 4 4
  spline S117 degree 2 poles (43.5887, 111.8299) (43.6276, 111.8299) (43.7106, 111.8247) (43.7884, 111.8118) (43.8506, 111.7936) (43.8688, 111.7806) knots 0 0 0 1 2 3 4 4 4
  line L197 (43.8688, 111.7806) -> (43.7287, 111.5291)
  spline S118 degree 2 poles (43.7287, 111.5291) (43.7183, 111.5291) (43.7002, 111.5317) knots 0 0 0 1 1 1
  spline S119 degree 2 poles (43.7002, 111.5317) (43.6872, 111.5343) (43.6509, 111.5368) (43.6276, 111.5368) knots 0 0 0 1 2 2 2
  spline S120 degree 2 poles (43.6276, 111.5368) (43.5394, 111.5368) (43.4434, 111.4539) (43.3967, 111.3086) (43.389, 111.1193) (43.389, 111.0155) knots 0 0 0 1 2 3 4 4 4
  line L198 (43.389, 111.0155) -> (43.389, 108.5906)
  spline S121 degree 2 poles (43.389, 108.5906) (43.389, 108.4868) (43.3967, 108.2975) (43.4434, 108.1523) (43.5394, 108.0693) (43.6276, 108.0693) knots 0 0 0 1 2 3 4 4 4
  spline S122 degree 2 poles (43.6276, 108.0693) (43.6509, 108.0693) (43.6872, 108.0719) (43.7002, 108.0719) knots 0 0 0 1 2 2 2
  spline S123 degree 2 poles (43.7002, 108.0719) (43.7183, 108.0745) (43.7287, 108.0797) knots 0 0 0 1 1 1
  line L199 (43.7287, 108.0797) -> (43.8688, 107.8255)
  spline S124 degree 2 poles (43.8688, 107.8255) (43.8506, 107.8151) (43.7884, 107.7944) (43.7106, 107.7814) (43.6276, 107.7762) (43.5887, 107.7762) knots 0 0 0 1 2 3 4 4 4
  spline S125 degree 2 poles (43.5887, 107.7762) (43.3838, 107.7762) (43.1452, 107.9033) (43.0233, 108.1315) (42.987, 108.4402) (42.987, 108.6191) knots 0 0 0 1 2 3 4 4 4
  line L200 (42.987, 108.6191) -> (42.987, 110.987)
  spline S126 degree 2 poles (45.5987, 108.5854) (45.4275, 108.5854) (45.1422, 108.7151) (44.9166, 108.9407) (44.7454, 109.2416) (44.6313, 109.5839) (44.5742, 109.947) (44.5742, 110.126) knots 0 0 0 1 2 3 4 5 6 6 6
  spline S127 degree 2 poles (44.5742, 110.126) (44.5742, 110.3049) (44.6235, 110.6758) (44.7272, 111.0155) (44.8906, 111.3138) (45.1163, 111.5343) (45.4119, 111.6639) (45.5987, 111.6639) knots 0 0 0 1 2 3 4 5 6 6 6
  spline S128 degree 2 poles (45.5987, 111.6639) (45.7698, 111.6639) (46.0551, 111.5343) (46.2808, 111.3086) (46.4519, 111.0078) (46.566, 110.6654) (46.6231, 110.2997) (46.6231, 110.126) knots 0 0 0 1 2 3 4 5 6 6 6
  spline S129 degree 2 poles (46.6231, 110.126) (46.6231, 109.9444) (46.5738, 109.5735) (46.4701, 109.2338) (46.3067, 108.9355) (46.081, 108.7151) (45.7828, 108.5854) (45.5987, 108.5854) knots 0 0 0 1 2 3 4 5 6 6 6
  spline S130 degree 2 poles (44.9918, 110.2115) (44.9918, 110.0948) (45.0073, 109.8147) (45.0566, 109.532) (45.1422, 109.2675) (45.2796, 109.06) (45.4793, 108.9355) (45.6142, 108.9355) knots 0 0 0 1 2 3 4 5 6 6 6
  spline S131 degree 2 poles (45.6142, 108.9355) (45.7361, 108.9355) (45.9202, 109.0289) (46.0525, 109.1923) (46.1355, 109.4076) (46.1848, 109.6513) (46.2055, 109.9133) (46.2055, 110.0378) knots 0 0 0 1 2 3 4 5 6 6 6
  spline S132 degree 2 poles (46.2055, 110.0378) (46.2055, 110.1545) (46.19, 110.4346) (46.1407, 110.7147) (46.0551, 110.9818) (45.9177, 111.1867) (45.718, 111.3112) (45.5831, 111.3112) knots 0 0 0 1 2 3 4 5 6 6 6
  spline S133 degree 2 poles (45.5831, 111.3112) (45.4612, 111.3112) (45.2771, 111.2178) (45.1448, 111.057) (45.0618, 110.8392) (45.0125, 110.5954) (44.9918, 110.336) (44.9918, 110.2115) knots 0 0 0 1 2 3 4 5 6 6 6
  spline S134 degree 2 poles (47.1755, 108.92) (47.1755, 108.9874) (47.2274, 109.1093) (47.3182, 109.2001) (47.4349, 109.2519) (47.5049, 109.2519) knots 0 0 0 1 2 3 4 4 4
  spline S135 degree 2 poles (47.5049, 109.2519) (47.5723, 109.2519) (47.6916, 109.2001) (47.7824, 109.1093) (47.8343, 108.9874) (47.8343, 108.92) knots 0 0 0 1 2 3 4 4 4
  spline S136 degree 2 poles (47.8343, 108.92) (47.8343, 108.8525) (47.7824, 108.7306) (47.6942, 108.6399) (47.5749, 108.5854) (47.5075, 108.5854) knots 0 0 0 1 2 3 4 4 4
  spline S137 degree 2 poles (47.5075, 108.5854) (47.4401, 108.5854) (47.3182, 108.6399) (47.2274, 108.7306) (47.1755, 108.8525) (47.1755, 108.92) knots 0 0 0 1 2 3 4 4 4
  line L201 (48.5112, 108.6191) -> (48.5112, 108.9563)
  spline S138 degree 2 poles (48.5112, 108.9563) (48.6072, 109.1093) (48.8302, 109.405) (49.0558, 109.6799) (49.2763, 109.9263) (49.3697, 110.0274) knots 0 0 0 1 2 3 4 4 4
  spline S139 degree 2 poles (49.3697, 110.0274) (49.4708, 110.1415) (49.6549, 110.3386) (49.7976, 110.5357) (49.8806, 110.738) (49.8806, 110.8573) knots 0 0 0 1 2 3 4 4 4
  spline S140 degree 2 poles (49.8806, 110.8573) (49.8806, 110.9533) (49.808, 111.1245) (49.6783, 111.249) (49.4967, 111.3242) (49.3878, 111.3242) knots 0 0 0 1 2 3 4 4 4
  spline S141 degree 2 poles (49.3878, 111.3242) (49.2659, 111.3242) (49.087, 111.2567) (48.9521, 111.1504) (48.8535, 111.0155) (48.812, 110.9455) knots 0 0 0 1 2 3 4 4 4
  line L202 (48.812, 110.9455) -> (48.5293, 111.0674)
  spline S142 degree 2 poles (48.5293, 111.0674) (48.5812, 111.1971) (48.7446, 111.4175) (48.9651, 111.5757) (49.2452, 111.6639) (49.4189, 111.6639) knots 0 0 0 1 2 3 4 4 4
  spline S143 degree 2 poles (49.4189, 111.6639) (49.6212, 111.6639) (49.9376, 111.5187) (50.1581, 111.2853) (50.2722, 110.987) (50.2722, 110.834) knots 0 0 0 1 2 3 4 4 4
  spline S144 degree 2 poles (50.2722, 110.834) (50.2722, 110.681) (50.1581, 110.4009) (49.9869, 110.1519) (49.7898, 109.9289) (49.7094, 109.8329) knots 0 0 0 1 2 3 4 4 4
  spline S145 degree 2 poles (49.7094, 109.8329) (49.6031, 109.711) (49.3956, 109.475) (49.2037, 109.2468) (49.0403, 109.0367) (48.9806, 108.9407) knots 0 0 0 1 2 3 4 4 4
  line L203 (48.9806, 108.9407) -> (50.3241, 108.9407)
  line L204 (50.3241, 108.9407) -> (50.3241, 108.6191)
  line L205 (50.3241, 108.6191) -> (48.5112, 108.6191)
  line L206 (52.9928, 109.2208) -> (52.6323, 109.2208)
  line L207 (52.6323, 109.2208) -> (52.6323, 108.6191)
  line L208 (52.6323, 108.6191) -> (52.2096, 108.6191)
  line L209 (52.2096, 108.6191) -> (52.2096, 109.2208)
  line L210 (52.2096, 109.2208) -> (51.014, 109.2208)
  line L211 (51.014, 109.2208) -> (51.014, 109.5632)
  line L212 (51.014, 109.5632) -> (51.9865, 111.6691)
  line L213 (51.9865, 111.6691) -> (52.3678, 111.6302)
  line L214 (52.3678, 111.6302) -> (51.5327, 109.8225)
  line L215 (51.5327, 109.8225) -> (51.3459, 109.5424)
  line L216 (51.3459, 109.5424) -> (52.2096, 109.5424)
  line L217 (52.2096, 109.5424) -> (52.2096, 110.3594)
  line L218 (52.2096, 110.3594) -> (52.6323, 110.3257)
  line L219 (52.6323, 110.3257) -> (52.6323, 109.5424)
  line L220 (52.6323, 109.5424) -> (53.0239, 109.5424)
  line L221 (53.0239, 109.5424) -> (52.9928, 109.2208)
  spline S146 degree 2 poles (54.6501, 111.6639) (54.8342, 111.6639) (55.1481, 111.5628) (55.3737, 111.376) (55.5034, 111.1063) (55.5034, 110.9377) knots 0 0 0 1 2 3 4 4 4
  spline S147 degree 2 poles (55.5034, 110.9377) (55.5034, 110.8184) (55.4333, 110.6343) (55.3114, 110.4891) (55.1532, 110.3698) (55.0651, 110.3179) knots 0 0 0 1 2 3 4 4 4
  spline S148 degree 2 poles (55.0651, 110.3179) (55.2129, 110.2504) (55.4489, 110.0793) (55.6123, 109.8666) (55.6979, 109.6021) (55.6979, 109.4413) knots 0 0 0 1 2 3 4 4 4
  spline S149 degree 2 poles (55.6979, 109.4413) (55.6979, 109.2208) (55.5215, 108.8966) (55.231, 108.6865) (54.8576, 108.5854) (54.6631, 108.5854) knots 0 0 0 1 2 3 4 4 4
  spline S150 degree 2 poles (54.6631, 108.5854) (54.4711, 108.5854) (54.1184, 108.6995) (53.8487, 108.9226) (53.6827, 109.2545) (53.6827, 109.4698) knots 0 0 0 1 2 3 4 4 4
  spline S151 degree 2 poles (53.6827, 109.4698) (53.6827, 109.6306) (53.7761, 109.8925) (53.9369, 110.1) (54.1573, 110.2634) (54.2844, 110.3257) knots 0 0 0 1 2 3 4 4 4
  spline S152 degree 2 poles (54.2844, 110.3257) (54.191, 110.3827) (54.0276, 110.5072) (53.9058, 110.6499) (53.8357, 110.8158) (53.8357, 110.9144) knots 0 0 0 1 2 3 4 4 4
  spline S153 degree 2 poles (53.8357, 110.9144) (53.8357, 111.1089) (53.9913, 111.3942) (54.2325, 111.5757) (54.5178, 111.6639) (54.6501, 111.6639) knots 0 0 0 1 2 3 4 4 4
  spline S154 degree 2 poles (54.6268, 110.1441) (54.4997, 110.0922) (54.2974, 109.96) (54.1547, 109.794) (54.0769, 109.5865) (54.0769, 109.4516) knots 0 0 0 1 2 3 4 4 4
  spline S155 degree 2 poles (54.0769, 109.4516) (54.0769, 109.3297) (54.1755, 109.1326) (54.3389, 108.99) (54.5515, 108.9148) (54.6631, 108.9148) knots 0 0 0 1 2 3 4 4 4
  spline S156 degree 2 poles (54.6631, 108.9148) (54.7927, 108.9148) (55.0236, 108.9848) (55.1973, 109.1223) (55.2985, 109.322) (55.2985, 109.4516) knots 0 0 0 1 2 3 4 4 4
  spline S157 degree 2 poles (55.2985, 109.4516) (55.2985, 109.5865) (55.1792, 109.7992) (54.9898, 109.9652) (54.7512, 110.0922) (54.6268, 110.1441) knots 0 0 0 1 2 3 4 4 4
  spline S158 degree 2 poles (54.7123, 110.4709) (54.8965, 110.5539) (55.1169, 110.7873) (55.1169, 110.9533) knots 0 0 0 1 2 2 2
  spline S159 degree 2 poles (55.1169, 110.9533) (55.1169, 111.0544) (55.0339, 111.1971) (54.9095, 111.2905) (54.7564, 111.332) (54.689, 111.332) knots 0 0 0 1 2 3 4 4 4
  spline S160 degree 2 poles (54.689, 111.332) (54.5982, 111.332) (54.4296, 111.2775) (54.3, 111.1763) (54.2222, 111.0415) (54.2222, 110.9611) knots 0 0 0 1 2 3 4 4 4
  spline S161 degree 2 poles (54.2222, 110.9611) (54.2222, 110.8677) (54.3, 110.7277) (54.4348, 110.6135) (54.6138, 110.515) (54.7123, 110.4709) knots 0 0 0 1 2 3 4 4 4
  line L222 (56.4345, 111.6302) -> (58.2396, 111.6302)
  line L223 (58.2396, 111.6302) -> (58.2396, 111.3683)
  spline S162 degree 2 poles (58.2396, 111.3683) (58.2396, 111.2827) (58.1099, 111.0129) (57.9102, 110.6758) (57.6716, 110.2868) (57.4563, 109.8796) (57.2955, 109.4698) (57.2722, 109.2805) knots 0 0 0 1 2 3 4 5 6 6 6
  spline S163 degree 2 poles (57.2722, 109.2805) (57.2618, 109.1975) (57.254, 109.0237) (57.2462, 108.8499) (57.2462, 108.7669) knots 0 0 0 1 2 3 3 3
  line L224 (57.2462, 108.7669) -> (57.2462, 108.6191)
  line L225 (57.2462, 108.6191) -> (56.8364, 108.6191)
  spline S164 degree 2 poles (56.8364, 108.6191) (56.8364, 108.6788) (56.8364, 108.8811) (56.8442, 109.1067) (56.8624, 109.3272) (56.8805, 109.405) knots 0 0 0 1 2 3 4 4 4
  spline S165 degree 2 poles (56.8805, 109.405) (56.9246, 109.6202) (57.0984, 110.0352) (57.3007, 110.419) (57.5134, 110.7614) (57.6871, 111.0389) (57.7961, 111.249) (57.7961, 111.3086) knots 0 0 0 1 2 3 4 5 6 6 6
  line L226 (57.7961, 111.3086) -> (56.4345, 111.3086)
  line L227 (56.4345, 111.3086) -> (56.4345, 111.6302)
  line L228 (59.2925, 111.6302) -> (59.2925, 111.4305)
  spline S166 degree 2 poles (59.2925, 111.4305) (59.2925, 111.3527) (59.264, 111.1297) (59.2484, 111.0207) knots 0 0 0 1 2 2 2
  spline S167 degree 2 poles (59.2484, 111.0207) (59.2277, 110.8962) (59.2043, 110.7614) knots 0 0 0 1 1 1
  line L229 (59.2043, 110.7614) -> (59.0306, 110.7614)
  spline S168 degree 2 poles (59.0306, 110.7614) (59.0072, 110.8962) (58.9865, 111.0207) knots 0 0 0 1 1 1
  spline S169 degree 2 poles (58.9865, 111.0207) (58.9709, 111.1297) (58.9424, 111.3527) (58.9424, 111.4305) knots 0 0 0 1 2 2 2
  line L230 (58.9424, 111.4305) -> (58.9424, 111.6302)
  line L231 (58.9424, 111.6302) -> (59.2925, 111.6302)
  line L232 (59.8968, 111.6302) -> (59.8968, 111.4305)
  spline S170 degree 2 poles (59.8968, 111.4305) (59.8968, 111.3527) (59.8683, 111.1297) (59.8527, 111.0207) knots 0 0 0 1 2 2 2
  spline S171 degree 2 poles (59.8527, 111.0207) (59.832, 110.8962) (59.8086, 110.7614) knots 0 0 0 1 1 1
  line L233 (59.8086, 110.7614) -> (59.6349, 110.7614)
  spline S172 degree 2 poles (59.6349, 110.7614) (59.6115, 110.8962) (59.5908, 111.0207) knots 0 0 0 1 1 1
  spline S173 degree 2 poles (59.5908, 111.0207) (59.5752, 111.1297) (59.5467, 111.3527) (59.5467, 111.4305) knots 0 0 0 1 2 2 2
  line L234 (59.5467, 111.4305) -> (59.5467, 111.6302)
  line L235 (59.5467, 111.6302) -> (59.8968, 111.6302)
  line L236 (61.7538, 110.8262) -> (62.0546, 110.8262)
  line L237 (62.0546, 110.8262) -> (62.0546, 111.1374)
  spline S174 degree 2 poles (62.0546, 111.1374) (62.0546, 111.3086) (62.1299, 111.5757) (62.2881, 111.7625) (62.5396, 111.8636) (62.716, 111.8636) knots 0 0 0 1 2 3 4 4 4
  spline S175 degree 2 poles (62.716, 111.8636) (62.8068, 111.8636) (62.9572, 111.8325) (63.0843, 111.7858) (63.1906, 111.721) (63.2321, 111.6873) knots 0 0 0 1 2 3 4 4 4
  line L238 (63.2321, 111.6873) -> (63.0609, 111.4487)
  spline S176 degree 2 poles (63.0609, 111.4487) (63.0194, 111.4798) (62.8716, 111.542) (62.7808, 111.542) knots 0 0 0 1 2 2 2
  spline S177 degree 2 poles (62.7808, 111.542) (62.6071, 111.542) (62.4255, 111.3475) (62.4255, 111.1167) knots 0 0 0 1 2 2 2
  line L239 (62.4255, 111.1167) -> (62.4255, 110.8262)
  line L240 (62.4255, 110.8262) -> (63.0091, 110.8262)
  line L241 (63.0091, 110.8262) -> (62.9676, 110.5046)
  line L242 (62.9676, 110.5046) -> (62.4359, 110.5046)
  line L243 (62.4359, 110.5046) -> (62.4359, 108.6191)
  line L244 (62.4359, 108.6191) -> (62.0546, 108.6191)
  line L245 (62.0546, 108.6191) -> (62.0546, 110.5046)
  line L246 (62.0546, 110.5046) -> (61.7538, 110.5046)
  line L247 (61.7538, 110.5046) -> (61.7538, 110.8262)
  spline S178 degree 2 poles (64.6067, 110.5228) (64.5263, 110.5228) (64.3681, 110.4579) (64.2228, 110.349) (64.0958, 110.2064) (64.0413, 110.126) knots 0 0 0 1 2 3 4 4 4
  line L248 (64.0413, 110.126) -> (64.0413, 108.6191)
  line L249 (64.0413, 108.6191) -> (63.66, 108.6191)
  line L250 (63.66, 108.6191) -> (63.66, 110.8288)
  line L251 (63.66, 110.8288) -> (64.0413, 110.8677)
  line L252 (64.0413, 110.8677) -> (64.0413, 110.4164)
  line L253 (64.0413, 110.4164) -> (64.241, 110.7692)
  spline S179 degree 2 poles (64.241, 110.7692) (64.2669, 110.7847) (64.3473, 110.8184) (64.4459, 110.8444) (64.56, 110.8625) (64.6222, 110.8625) knots 0 0 0 1 2 3 4 4 4
  spline S180 degree 2 poles (64.6222, 110.8625) (64.713, 110.8625) (64.8349, 110.8314) (64.8634, 110.8158) knots 0 0 0 1 2 2 2
  line L254 (64.8634, 110.8158) -> (64.8453, 110.4839)
  spline S181 degree 2 poles (64.8453, 110.4839) (64.8142, 110.4916) (64.6949, 110.5228) (64.6067, 110.5228) knots 0 0 0 1 2 2 2
  spline S182 degree 2 poles (66.0643, 108.5854) (65.8412, 108.5854) (65.4755, 108.7592) (65.211, 109.0678) (65.0631, 109.4879) (65.0631, 109.7291) knots 0 0 0 1 2 3 4 4 4
  spline S183 degree 2 poles (65.0631, 109.7291) (65.0631, 109.9729) (65.2032, 110.3879) (65.4651, 110.6914) (65.836, 110.8625) (66.0643, 110.8625) knots 0 0 0 1 2 3 4 4 4
  spline S184 degree 2 poles (66.0643, 110.8625) (66.2873, 110.8625) (66.6582, 110.6914) (66.9227, 110.3879) (67.0705, 109.9729) (67.0705, 109.7291) knots 0 0 0 1 2 3 4 4 4
  spline S185 degree 2 poles (67.0705, 109.7291) (67.0705, 109.4879) (66.9279, 109.0678) (66.666, 108.7592) (66.2925, 108.5854) (66.0643, 108.5854) knots 0 0 0 1 2 3 4 4 4
  spline S186 degree 2 poles (66.6893, 109.6747) (66.6893, 109.8381) (66.6193, 110.1519) (66.4663, 110.3983) (66.2251, 110.5513) (66.0565, 110.5513) knots 0 0 0 1 2 3 4 4 4
  spline S187 degree 2 poles (66.0565, 110.5513) (65.8957, 110.5513) (65.6623, 110.419) (65.5144, 110.1986) (65.4444, 109.9159) (65.4444, 109.7681) knots 0 0 0 1 2 3 4 4 4
  spline S188 degree 2 poles (65.4444, 109.7681) (65.4444, 109.6047) (65.5144, 109.2934) (65.6649, 109.047) (65.9035, 108.8966) (66.072, 108.8966) knots 0 0 0 1 2 3 4 4 4
  spline S189 degree 2 poles (66.072, 108.8966) (66.2302, 108.8966) (66.4637, 109.0289) (66.6167, 109.2493) (66.6893, 109.5294) (66.6893, 109.6747) knots 0 0 0 1 2 3 4 4 4
  line L255 (68.0561, 108.6191) -> (67.6748, 108.6191)
  line L256 (67.6748, 108.6191) -> (67.6748, 110.8288)
  line L257 (67.6748, 110.8288) -> (68.0561, 110.8677)
  line L258 (68.0561, 110.8677) -> (68.0561, 110.4994)
  line L259 (68.0561, 110.4994) -> (68.178, 110.7147)
  spline S190 degree 2 poles (68.178, 110.7147) (68.2143, 110.7406) (68.3232, 110.7925) (68.4607, 110.834) (68.6163, 110.8625) (68.6993, 110.8625) knots 0 0 0 1 2 3 4 4 4
  spline S191 degree 2 poles (68.6993, 110.8625) (68.9223, 110.8625) (69.205, 110.6421) (69.2465, 110.4735) knots 0 0 0 1 2 2 2
  line L260 (69.2465, 110.4735) -> (69.3995, 110.7069)